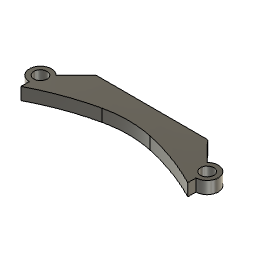
Finger1Section1P1V1 v3 (Autodesk Fusion 360 design; units mm, degrees)
Autodesk Fusion 360 part; units mm, degrees
sketch "Sketch1" plane through (0, 0, 0) normal (0, 0, 1) x (1, 0, 0)
  circle A0 centre (0.507, 0) radius 1.2
  line L0 (4.507, 4) -> (5.507, 5)
  arc A1 (1.9212, 1.4142) -> (0.507, -2) centre (0.507, 0) ccw
  line L1 (1.9212, 1.4142) -> (4.507, 4)
  line L2 (0.507, -2) -> (0.507, -3.5)
  line L3 (5.507, 5) -> (15.5594, 5)
  line L4 (25.5594, 5) -> (25.6118, 5)
  arc A2 (11.1884, 0.3961) -> (0.507, -3.5) centre (20.507, -41.7412) ccw
  arc A3 (30.507, -2) -> (29.0928, 1.4142) centre (30.507, 0) ccw
  line L5 (25.6118, 5) -> (26.507, 4)
  arc A4 (30.507, -3.5) -> (19.8257, 0.3961) centre (10.507, -41.7412) ccw
  line L6 (30.507, -2) -> (30.507, -3.5)
  line L7 (15.5594, 1.1297) -> (15.5594, 1.1174)
  line L8 (15.5594, 5) -> (25.6118, 5)
  line L9 (29.0928, 1.4142) -> (26.507, 4)
  circle A5 centre (30.507, 0) radius 1.2
  arc A6 (19.8257, 0.3961) -> (11.1884, 0.3961) centre (15.507, -19.1321) ccw
  dimension "d3" = 2.4
  dimension "d7" = 4
  dimension "d10" = 1.5
  dimension "d16" = 2.4
  dimension "d17" = 4
  dimension "d18" = 1.5
  dimension "d19" = 20
  constraint concentric A0 A1
  constraint coincident L4.start L3
  constraint collinear L3 L4
  constraint coincident L7.start A2
  constraint coincident L7.end A4
  constraint tangent A2 A6
  constraint tangent A4 A6
  measures "d3" diameter of A0
  measures "d7" diameter of A1
  measures "d10" distance of L2.end A1.end
  measures "d16" diameter of A5
  measures "d17" diameter of A3
  measures "d18" distance of A3.start A4.start
  measures "d19" radius of A6
extrude "Extrude2" add sketch "Sketch1" along normal blind 2.2
